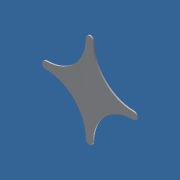
# Autodesk Inventor part: Podstawa
Saved by Autodesk Inventor 2014 SP1 (Build 180222100, 222)
## iProperties
Created: 2014-08-30
Part Number: Podstawa
Material: Tworzywo sztuczne ABS
Document SubType Name: Modeling
Designer: Marcin
Density: 1.06 g/cm^3
Appearance: Gładkie - białe
Author: Marcin
Autodesk Inventor part; units mm, degrees
ref_plane "YZ Plane" through (0, 0, 0) normal (1, 0, 0) x (0, 1, 0)
ref_plane "XZ Plane" through (0, 0, 0) normal (0, 1, 0) x (-1, 0, 0)
ref_plane "XY Plane" through (0, 0, 0) normal (0, 0, 1) x (1, 0, 0)
sketch "Szkic1" plane through (0, 0, 0) normal (0, 1, 0) x (-1, 0, 0)
  line L0 (0, 0) -> (0, -135)
  line L1 (0, 0) -> (-135, 0)
  arc A0 (-10, -125) -> (0, -135) centre (0, -125) ccw
  arc A1 (-135, 0) -> (-125, -10) centre (-125, 0) ccw
  arc A2 (-10, -125) -> (-125, -10) centre (-125, -125) ccw
  line L2 (0, 0) -> (135, 0)
  arc A3 (0, -135) -> (10, -125) centre (0, -125) ccw
  arc A4 (125, -10) -> (135, 0) centre (125, 0) ccw
  arc A5 (125, -10) -> (10, -125) centre (125, -125) ccw
  line L3 (0, 0) -> (0, 135)
  arc A6 (0, 135) -> (-10, 125) centre (0, 125) ccw
  arc A7 (-125, 10) -> (-135, 0) centre (-125, 0) ccw
  arc A8 (-125, 10) -> (-10, 125) centre (-125, 125) ccw
  arc A9 (10, 125) -> (0, 135) centre (0, 125) ccw
  arc A10 (135, 0) -> (125, 10) centre (125, 0) ccw
  arc A11 (10, 125) -> (125, 10) centre (125, 125) ccw
  circle A12 centre (-127, 0) radius 2.5
  circle A13 centre (-76, 0) radius 2.5
  circle A14 centre (0, 127) radius 2.5
  circle A15 centre (0, 76) radius 2.5
  circle A16 centre (0, -127) radius 2.5
  circle A17 centre (0, -76) radius 2.5
  circle A18 centre (127, 0) radius 2.5
  circle A19 centre (76, 0) radius 2.5
  dimension "d13" = 135
  dimension "d14" = 135
  dimension "d15" = 20
  dimension "d16" = 20
  dimension "d17" = 115
  dimension "d18" = 125
  dimension "sruba" = 5
  dimension "d20" = 8
  dimension "d21" = 5
  dimension "d22" = 51
  dimension "d23" = 5
  dimension "d24" = 5
  dimension "d25" = 8
  dimension "d26" = 51
  constraints: 24 point on circle, 20 centre point, 17 symmetric about line, 8 end point, 8 point on line, 1 perpendicular, 1 tangent, 1 vertical, 14 other
  measures "d13" distance of L0.start L0.end
  measures "d14" distance of L0.start L1.end
  measures "d15" diameter of A0
  measures "d16" diameter of A1
  measures "d17" radius of A2
  measures "d18" distance from line of L1 A0.start
  measures "sruba" diameter of A12
  measures "d20" distance of A12.centre L1.end
  measures "d21" diameter of A13
  measures "d22" distance of A13.centre A12.centre
  measures "d23" diameter of A14
  measures "d24" diameter of A15
  measures "d25" distance of L3.end A14.centre
  measures "d26" distance of A14.centre A15.centre
extrude "Wyciągnięcie proste1" add sketch "Szkic1" along normal blind 3.74
equation "\"d14\" = d13"
equation "\"d16\" = d15"
equation "\"d21\" = sruba"
equation "\"d23\" = sruba"
equation "\"d24\" = sruba"
equation "\"d25\" = d20"
equation "\"d26\" = d22"
